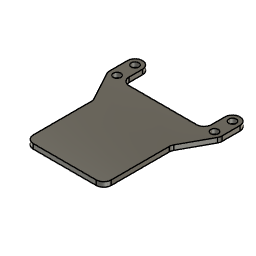
Tray v6 (Autodesk Fusion 360 design; units mm, degrees)
Autodesk Fusion 360 part; units mm, degrees
sketch "Sketch1" plane through (0, 0, 0) normal (0, 0, 1) x (1, 0, 0)
  circle A0 centre (0, 0) radius 2.5
  circle A1 centre (0, 12) radius 2.5
  circle A2 centre (65, 0) radius 2.5
  circle A3 centre (0, 12) radius 5
  line L0 (5, -2) -> (60, -2)
  line L1 (5, 12) -> (5, -2)
  circle A4 centre (0, 0) radius 5
  line L2 (-5, 0) -> (-5, 12)
  line L3 (0, 0) -> (65, 0) construction
  line L4 (32.5, 0) -> (32.5, -19.0435) construction
  line L5 (4.5, -9.5218) -> (60.5, -9.5218) construction
  line L6 (-4.3911, -2.3912) -> (6.5, -22.3912)
  line L7 (6.5, -22.3912) -> (6.5, -67.3912)
  line L8 (6.5, -67.3912) -> (32.5, -67.3912)
  line L9 (58.5, -67.3912) -> (32.5, -67.3912)
  line L10 (58.5, -22.3912) -> (58.5, -67.3912)
  line L11 (69.3911, -2.3912) -> (58.5, -22.3912)
  circle A5 centre (65, 0) radius 5
  line L12 (70, 0) -> (70, 12)
  circle A6 centre (65, 12) radius 5
  line L13 (60, 12) -> (60, -2)
  circle A7 centre (65, 12) radius 2.5
  dimension "d1" = 5
  dimension "d2" = 5
  dimension "d3" = 5
  dimension "d5" = 12
  dimension "d6" = 65
  dimension "d9" = 2
  dimension "d10" = 10
  dimension "d12" = 56
  dimension "d13" = 45
  dimension "d14" = 26
  dimension "d15" = 20
  constraint coincident A0.centre A4.centre
  constraint vertical A0.centre A1.centre
  constraint horizontal A0.centre A2.centre
  constraint concentric A1 A3
  constraint horizontal L0
  constraint coincident A3 L1.start
  constraint perpendicular L0 L1
  constraint tangent A3 L1
  constraint coincident L0 L1.end
  constraint coincident A4 L2.start
  constraint coincident A3 L2.end
  constraint tangent A3 L2
  constraint vertical L2
  constraint coincident A2.centre L3.end
  constraint midpoint L3 L4.start
  constraint perpendicular L3 L4
  constraint parallel L0 L5
  constraint midpoint L4 L5
  constraint coincident A4 L6.start
  constraint tangent A4 L6
  constraint vertical L7
  constraint perpendicular L7 L8
  constraint vertical L4.end L8.end
  constraint symmetric A1 L4 A7
  constraint symmetric A3 L4 A6
  constraint symmetric L1.start L4 L13.start
  constraint symmetric L0.start L4 L0.end
  constraint symmetric A4 L4 A5
  constraint symmetric L2.start L4 L12.start
  constraint symmetric L2.end L4 L12.end
  constraint symmetric L4 L6.start L11.start
  constraint symmetric L4 L6.end L10.start
  constraint symmetric L4 L7.end L9.start
  constraint symmetric L4 L8.end L9.end
  constraint coincident L0.start L1.end
  constraint coincident L0.end L13.end
  measures "d1" diameter of A0
  measures "d2" diameter of A1
  measures "d3" diameter of A2
  measures "d5" distance of A0.centre A1.centre
  measures "d6" distance of A0.centre A2.centre
  measures "d9" distance of A0.centre L0
  measures "d10" diameter of A4
  measures "d12" distance of L5.start L5.end
  measures "d13" distance of L6.end L7.end
  measures "d14" distance of L7.end L8.end
  measures "d15" vertical distance of L6.start L6.end
extrude "Extrude1" add sketch "Sketch1" along normal blind 3.175
fillet "Fillet1" radius 5 6 edges at (5, -2, 1.5875) (60, -2, 1.5875) (58.5, -67.3912, 1.5875) (6.5, -67.3912, 1.5875) (58.5, -22.3912, 1.5875) (6.5, -22.3912, 1.5875)
